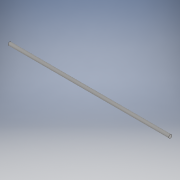
# Autodesk Inventor part: T8LeadScrew
Saved by Autodesk Inventor 2018 (Build 220112000, 112)
## iProperties
Created: 2017-10-01
Part Number: T8LeadScrew
Material: Generic
Document SubType Name: Modeling
Designer: Jurjen
Density: 1 g/cm^3
Appearance: Default
Author: Jurjen
Autodesk Inventor part; units mm, degrees
ref_plane "YZ Plane" through (0, 0, 0) normal (1, 0, 0) x (0, 1, 0)
ref_plane "XZ Plane" through (0, 0, 0) normal (0, 1, 0) x (-1, 0, 0)
ref_plane "XY Plane" through (0, 0, 0) normal (0, 0, 1) x (1, 0, 0)
sketch "Sketch1" plane through (0, 0, 0) normal (0, 1, 0) x (-1, 0, 0)
  line L0 (200, 0) -> (-200, 0)
  line L1 (-200, 0) -> (-200, -4)
  line L2 (-200, -4) -> (200, -4)
  line L3 (200, -4) -> (200, 0)
  point P0 (0, 0)
  point P1 (0, -4)
  point P2 (0, 0)
  dimension "d0" = 4
  dimension "d1" = 400
  constraints: 8 end point, 2 midpoint, 2 parallel, 1 horizontal, 1 horizontal alignment, 1 perpendicular, 1 vertical alignment
  measures "d0" distance between parallel lines of L0 L2
  measures "d1" distance of L1.end L2.end
revolve "Revolution1" add sketch "Sketch1" angle 360 about axis through (-200, 0, 0) along (1, 0, 0)
thread "Thread1" size "M8x1.25" class "6g" standard "ISO Metric profile" full length
body "Solid1"
